Autodesk Fusion 360 part; units mm, degrees
(part 2 of 2)
  spline S52 degree 3 poles (338.481, 94.0744) (339.0332, 94.0744) (339.4811, 94.5223) (339.4811, 95.0745) knots 0 0 0 0 1 1 1 1
  line L284 (337.981, 116.5126) -> (323.981, 116.5126)
  line L285 (321.3125, 131.0875) -> (321.3125, 145.0875)
  line L286 (135.8625, 73.9375) -> (149.8625, 73.9375)
  spline S53 degree 3 poles (90.6256, 72.4374) (91.1779, 72.4374) (91.6256, 72.8853) (91.6256, 73.4375) knots 0 0 0 0 1 1 1 1
  line L287 (302.2625, 54.8875) -> (302.2625, 68.8875)
  spline S54 degree 3 poles (140.6067, 54.8919) (141.159, 54.8919) (141.6067, 55.3398) (141.6067, 55.892) knots 0 0 0 0 1 1 1 1
  line L288 (323.481, 117.9507) -> (338.481, 117.9507)
  line L289 (159.3875, 126.0375) -> (145.3875, 126.0375)
  line L290 (121.2875, 126.0375) -> (107.2875, 126.0375)
  line L291 (111.7625, 131.0875) -> (111.7625, 145.0875)
  line L292 (73.6625, 145.0875) -> (59.6625, 145.0875)
  line L293 (59.6625, 131.0875) -> (73.6625, 131.0875)
  line L294 (62.0435, 54.8875) -> (76.0435, 54.8875)
  line L295 (207.0125, 131.0875) -> (207.0125, 145.0875)
  line L296 (169.2005, 92.9875) -> (183.2005, 92.9875)
  line L297 (254.6375, 126.0375) -> (240.6375, 126.0375)
  spline S55 degree 3 poles (82.0506, 61.8875) (82.0506, 61.28) (81.5581, 60.7875) (80.9506, 60.7875) (80.3431, 60.7875) (79.8506, 61.28) (79.8506, 61.8875) (79.8506, 62.495) (80.3431, 62.9875) (80.9506, 62.9875) (81.5581, 62.9875) (82.0506, 62.495) (82.0506, 61.8875) knots 0 0 0 0 1 1 1 2 2 2 3 3 3 4 4 4 4
  line L298 (234.6062, 55.892) -> (234.6062, 69.392)
  line L299 (80.8065, 106.9875) -> (66.8065, 106.9875)
  line L300 (116.8125, 87.9375) -> (116.8125, 73.9375)
  line L301 (202.5375, 112.0375) -> (216.5375, 112.0375)
  line L302 (168.9125, 87.9375) -> (154.9125, 87.9375)
  line L303 (212.0625, 87.9375) -> (212.0625, 73.9375)
  line L304 (187.9625, 87.9375) -> (173.9625, 87.9375)
  line L305 (126.0505, 106.9875) -> (112.0505, 106.9875)
  line L306 (130.8125, 87.9375) -> (116.8125, 87.9375)
  line L307 (337.981, 102.5126) -> (337.981, 116.5126)
  line L308 (226.0625, 131.0875) -> (226.0625, 145.0875)
  line L309 (212.0625, 131.0875) -> (226.0625, 131.0875)
extrude "拉伸2" add sketch "草图2" along normal blind 1.5
